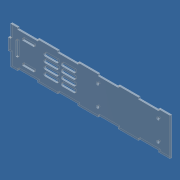
# Autodesk Inventor part: Top
Saved by Autodesk Inventor 2016 (Build 200138000, 138)
## iProperties
Created: 2016-04-03
Part Number: Top
Material: Polycarbonate, Clear
Document SubType Name: Modeling
Designer: admin
Density: 1.2 g/cm^3
Appearance: Polycarbonate - Clear
Author: admin
Autodesk Inventor part; units mm, degrees
ref_plane "YZ Plane" through (0, 0, 0) normal (1, 0, 0) x (0, 1, 0)
ref_plane "XZ Plane" through (0, 0, 0) normal (0, 1, 0) x (-1, 0, 0)
ref_plane "XY Plane" through (0, 0, 0) normal (0, 0, 1) x (1, 0, 0)
derived "Wall.ipt"
sketch "Sketch1" plane through (0, 0, 0) normal (0, 0, 1) x (1, 0, 0)
  line L0 (142.5, -22.5) -> (142.5, 22.5)
  line L1 (142.5, 22.5) -> (-137.5, 22.5)
  arc A0 (-169.3198, -9.3198) -> (-157.5, -22.5) centre (-130.5627, 13.547) ccw
  line L2 (-154.4706, 5.5294) -> (-150.935, 1.9939)
  line L3 (-150.935, 1.9939) -> (-152.2157, 0.7132)
  line L4 (-152.2157, 0.7132) -> (-150.8015, -0.701)
  line L5 (-150.8015, -0.701) -> (-149.5208, 0.5797)
  line L6 (-149.5208, 0.5797) -> (-147.3995, -1.5416)
  line L7 (-147.3995, -1.5416) -> (-145.2782, 0.5797)
  line L8 (-145.2782, 0.5797) -> (-147.3995, 2.701)
  line L9 (-147.3995, 2.701) -> (-146.1188, 3.9817)
  line L10 (-146.1188, 3.9817) -> (-147.533, 5.3959)
  line L11 (-147.533, 5.3959) -> (-148.8137, 4.1152)
  line L12 (-148.8137, 4.1152) -> (-152.3492, 7.6508)
  line L13 (-154.542, 7.7222) -> (-156.666, 9.8462) construction
  line L14 (-122.5, 22.5) -> (-122.5, 25.5)
  line L15 (-122.5, 25.5) -> (-87.5, 25.5)
  line L16 (-87.5, 25.5) -> (-87.5, 22.5)
  line L17 (-52.5, 22.5) -> (-52.5, 25.5)
  line L18 (-52.5, 25.5) -> (-17.5, 25.5)
  line L19 (-17.5, 25.5) -> (-17.5, 22.5)
  line L20 (17.5, 22.5) -> (17.5, 25.5)
  line L21 (17.5, 25.5) -> (52.5, 25.5)
  line L22 (52.5, 25.5) -> (52.5, 22.5)
  line L23 (87.5, 22.5) -> (87.5, 25.5)
  line L24 (87.5, 25.5) -> (122.5, 25.5)
  line L25 (122.5, 25.5) -> (122.5, 22.5)
  line L26 (87.5, 22.5) -> (52.5, 22.5)
  line L27 (-52.5, 22.5) -> (-87.5, 22.5)
  line L28 (-122.5, 22.5) -> (-137.5, 22.5)
  line L29 (-122.5, -22.5) -> (-122.5, -25.5)
  line L30 (-122.5, -25.5) -> (-87.5, -25.5)
  line L31 (-87.5, -25.5) -> (-87.5, -22.5)
  line L32 (-52.5, -22.5) -> (-52.5, -25.5)
  line L33 (-52.5, -25.5) -> (-17.5, -25.5)
  line L34 (-17.5, -25.5) -> (-17.5, -22.5)
  line L35 (17.5, -22.5) -> (17.5, -25.5)
  line L36 (17.5, -25.5) -> (52.5, -25.5)
  line L37 (52.5, -25.5) -> (52.5, -22.5)
  line L38 (87.5, -22.5) -> (87.5, -25.5)
  line L39 (87.5, -25.5) -> (122.5, -25.5)
  line L40 (122.5, -25.5) -> (122.5, -22.5)
  line L41 (-157.5, -22.5) -> (-122.5, -22.5)
  line L42 (-87.5, -22.5) -> (-52.5, -22.5)
  line L43 (-17.5, -22.5) -> (17.5, -22.5)
  line L44 (52.5, -22.5) -> (87.5, -22.5)
  line L45 (122.5, -22.5) -> (142.5, -22.5)
  line L46 (-1.5, 12.5) -> (-1.5, 22.5)
  line L47 (1.5, 22.5) -> (1.5, 12.5)
  line L48 (1.5, 12.5) -> (-1.5, 12.5)
  line L49 (-37.337, 0) -> (-30.889, 0) construction
  line L50 (-164.0165, -4.0165) -> (-166.1378, -1.8952)
  line L51 (-166.1378, -1.8952) -> (-161.8952, 2.3475)
  line L52 (-161.8952, 2.3475) -> (-159.7739, 0.2261)
  line L53 (-147.0459, 12.9541) -> (-149.1673, 15.0754)
  line L54 (-149.1673, 15.0754) -> (-144.9246, 19.318)
  line L55 (-144.9246, 19.318) -> (-142.8033, 17.1967)
  line L56 (-154.4706, 5.5294) -> (-159.7739, 0.2261)
  line L57 (-164.0165, -4.0165) -> (-169.3198, -9.3198)
  line L58 (-137.5, 22.5) -> (-142.8033, 17.1967)
  line L59 (-147.0459, 12.9541) -> (-152.3492, 7.6508)
  line L60 (17.5, 22.5) -> (1.5, 22.5)
  line L61 (-1.5, 22.5) -> (-17.5, 22.5)
  line L62 (131, 22.5) -> (131, 12.5)
  line L63 (131, 12.5) -> (134, 12.5)
  line L64 (134, 12.5) -> (134, 22.5)
  line L65 (122.5, 22.5) -> (131, 22.5)
  line L66 (134, 22.5) -> (142.5, 22.5)
  point P0 (0, 0)
  point P1 (142.5, 0)
  point P2 (-146.3388, -0.481)
  point P3 (2.493, 0)
  point P4 (0, -22.5)
  point P5 (1.5, -22.5)
sketch "Sketch2" plane through (0, 0, 0) normal (0, 1, 0) x (-1, 0, 0)
  line L0 (-142.5, 0) -> (137.5, 0) construction
  line L1 (-142.5, -65) -> (-142.5, 0)
  line L2 (134.5, -42.5) -> (138.5, -42.5)
  line L3 (138.5, -42.5) -> (138.5, -22.5)
  line L4 (138.5, -22.5) -> (134.5, -22.5)
  line L5 (134.5, 0) -> (134.5, -22.5)
  line L6 (134.5, -42.5) -> (134.5, -65)
  line L7 (122.5, 0) -> (122.5, -3)
  line L8 (122.5, -3) -> (87.5, -3)
  line L9 (87.5, -3) -> (87.5, 0)
  line L10 (52.5, 0) -> (52.5, -3)
  line L11 (52.5, -3) -> (17.5, -3)
  line L12 (17.5, -3) -> (17.5, 0)
  line L13 (-17.5, 0) -> (-17.5, -3)
  line L14 (-17.5, -3) -> (-52.5, -3)
  line L15 (-52.5, -3) -> (-52.5, 0)
  line L16 (-87.5, 0) -> (-87.5, -3)
  line L17 (-87.5, -3) -> (-122.5, -3)
  line L18 (-122.5, -3) -> (-122.5, 0)
  line L19 (122.5, -65) -> (122.5, -62)
  line L20 (122.5, -62) -> (87.5, -62)
  line L21 (87.5, -62) -> (87.5, -65)
  line L22 (52.5, -65) -> (52.5, -62)
  line L23 (17.5, -62) -> (17.5, -65)
  line L24 (17.5, -62) -> (52.5, -62)
  line L25 (-17.5, -65) -> (-17.5, -62)
  line L26 (-52.5, -62) -> (-52.5, -65)
  line L27 (-52.5, -62) -> (-17.5, -62)
  line L28 (-87.5, -65) -> (-87.5, -62)
  line L29 (-87.5, -62) -> (-122.5, -62)
  line L30 (-122.5, -62) -> (-122.5, -65)
  line L31 (134.5, -65) -> (122.5, -65)
  line L32 (87.5, -65) -> (52.5, -65)
  line L33 (17.5, -65) -> (-17.5, -65)
  line L34 (-52.5, -65) -> (-87.5, -65)
  line L35 (-122.5, -65) -> (-142.5, -65)
  line L36 (87.5, 0) -> (52.5, 0)
  line L37 (17.5, 0) -> (-17.5, 0)
  line L38 (-52.5, 0) -> (-87.5, 0)
  line L39 (-122.5, 0) -> (-142.5, 0)
  line L40 (134.5, 0) -> (122.5, 0)
  point P0 (0, 0)
  point P1 (138.5, -32.5)
  point P2 (-142.5, -32.5)
  dimension "d1" = 65
  dimension "d4" = 20
  dimension "d5" = 4
  dimension "d6" = 3
  dimension "d7" = 3
  constraints: 80 end point, 28 point on line, 25 perpendicular, 6 collinear, 6 horizontal, 4 vertical, 3 parallel, 2 midpoint, 1 horizontal alignment, 2 other
  measures "d1" distance of L1.start L1.end
  measures "d4" distance between parallel lines of L4 L2
  measures "d5" distance between parallel lines of L6 L3
  measures "d6" distance of L20.end L21.end
  measures "d7" distance from line of L5 point (137.5, 0)
extrude "Extrusion1" add sketch "Sketch2" along normal blind 3
sketch "Sketch4" plane through (0, 3, 0) normal (0, 1, 0) x (1, 0, 0)
  line L0 (-122.5, 45) -> (-125.5, 45)
  line L1 (-125.5, 45) -> (-125.5, 20)
  line L2 (-125.5, 20) -> (-122.5, 20)
  line L3 (-122.5, 20) -> (-122.5, 45)
  line L4 (142.5, 0) -> (142.5, 65) projected
  line L5 (142.5, 65) -> (122.5, 65) projected
  line L6 (122.5, 65) -> (122.5, 62) projected
  line L7 (122.5, 62) -> (87.5, 62) projected
  line L8 (87.5, 62) -> (87.5, 65) projected
  line L9 (87.5, 65) -> (52.5, 65) projected
  line L10 (52.5, 65) -> (52.5, 62) projected
  line L11 (52.5, 62) -> (17.5, 62) projected
  line L12 (17.5, 62) -> (17.5, 65) projected
  line L13 (17.5, 65) -> (-17.5, 65) projected
  line L14 (-17.5, 65) -> (-17.5, 62) projected
  line L15 (-17.5, 62) -> (-52.5, 62) projected
  line L16 (-52.5, 62) -> (-52.5, 65) projected
  line L17 (-52.5, 65) -> (-87.5, 65) projected
  line L18 (-87.5, 65) -> (-87.5, 62) projected
  line L19 (-87.5, 62) -> (-122.5, 62) projected
  line L20 (-122.5, 62) -> (-122.5, 65) projected
  line L21 (-122.5, 65) -> (-134.5, 65) projected
  line L22 (-134.5, 65) -> (-134.5, 42.5) projected
  line L23 (-134.5, 42.5) -> (-138.5, 42.5) projected
  line L24 (-138.5, 42.5) -> (-138.5, 22.5) projected
  line L25 (-138.5, 22.5) -> (-134.5, 22.5) projected
  line L26 (-134.5, 22.5) -> (-134.5, 0) projected
  line L27 (-134.5, 0) -> (-122.5, 0) projected
  line L28 (-122.5, 0) -> (-122.5, 3) projected
  line L29 (-122.5, 3) -> (-87.5, 3) projected
  line L30 (-87.5, 3) -> (-87.5, 0) projected
  line L31 (-87.5, 0) -> (-52.5, 0) projected
  line L32 (-52.5, 0) -> (-52.5, 3) projected
  line L33 (-52.5, 3) -> (-17.5, 3) projected
  line L34 (-17.5, 3) -> (-17.5, 0) projected
  line L35 (-17.5, 0) -> (17.5, 0) projected
  line L36 (17.5, 0) -> (17.5, 3) projected
  line L37 (17.5, 3) -> (52.5, 3) projected
  line L38 (52.5, 3) -> (52.5, 0) projected
  line L39 (52.5, 0) -> (87.5, 0) projected
  line L40 (87.5, 0) -> (87.5, 3) projected
  line L41 (87.5, 3) -> (122.5, 3) projected
  line L42 (122.5, 3) -> (122.5, 0) projected
  line L43 (122.5, 0) -> (142.5, 0) projected
  line L44 (-122.5, 62) -> (-122.5, 65) projected
  line L45 (-119.5, 86.0571) -> (-119.5, -26.187) construction
  line L46 (-117, 86.0571) -> (-117, -26.187) construction
  line L47 (-114, 53.2887) -> (-114, 7.6341) construction
  line L48 (-114, 53) -> (-94, 53)
  line L49 (-94, 53) -> (-94, 50)
  line L50 (-94, 50) -> (-114, 50)
  line L51 (-114, 50) -> (-114, 53)
  line L52 (-114, 15) -> (-94, 15)
  line L53 (-94, 15) -> (-94, 12)
  line L54 (-94, 12) -> (-114, 12)
  line L55 (-114, 12) -> (-114, 15)
  line L56 (-94.6514, 32.5) -> (-74.3553, 32.5) construction
  point P0 (0, 0)
  point P1 (-138.5, 32.5)
  point P2 (-122.5, 32.5)
  dimension "d20" = 25
  dimension "d24" = 265
  dimension "d25" = 3
  dimension "d27" = 2.5
  dimension "d28" = 3
  dimension "d29" = 35
  dimension "d30" = 20
  constraints: 32 end point, 6 parallel, 4 horizontal, 3 collinear, 3 equal length, 3 horizontal alignment, 3 perpendicular, 3 vertical, 2 midpoint, 1 point on line, 1 other
  measures "d20" distance between parallel lines of L2 L0
  measures "d24" distance between parallel lines of L4 L3
  measures "d25" distance between parallel lines of L45 L3
  measures "d27" distance between parallel lines of L45 L46
  measures "d28" distance between parallel lines of L47 L46
  measures "d29" distance between parallel lines of L52 L50
  measures "d30" distance of L53.end L54.end
extrude "Extrusion3" cut sketch "Sketch4" against normal up to next contours L3 L2 L1 L0 | L48 L49 L50 L51 | L52 L53 L54 L55
sketch "Sketch3" plane through (0, 3, 0) normal (0, 1, 0) x (1, 0, 0)
  arc A0 (-74.5, 19.5) -> (-74.5, 14.5) centre (-74.5, 17) ccw
  arc A1 (-54.5, 14.5) -> (-54.5, 19.5) centre (-54.5, 17) ccw
  line L0 (-74.5, 19.5) -> (-54.5, 19.5)
  line L1 (-74.5, 14.5) -> (-54.5, 14.5)
  line L2 (-122.5, 3) -> (-87.5, 3) projected
  line L3 (-134.5, 22.5) -> (-134.5, 0) projected
  point P0 (0, 0)
  dimension "d8" = 5
  dimension "d9" = 20
  dimension "d10" = 14
  dimension "d11" = 60
  constraints: 4 end point, 4 point on circle, 3 tangent, 2 centre point, 1 equal radius, 1 horizontal, 1 horizontal alignment
  measures "d8" diameter of A0
  measures "d9" distance of A1.centre A0.centre
  measures "d10" distance from line of L2 A0.centre
  measures "d11" distance from line of L3 A0.centre
extrude "Extrusion2" cut sketch "Sketch3" against normal blind 3
pattern_linear "Rectangular Pattern1" count 2 spacing 30 along (1, 0, 0) count 4 spacing 10 along (0, 0, -1) of "Extrusion2"
sketch "Sketch5" plane through (0, 0, 0) normal (0, -1, 0) x (1, 0, 0)
  line L0 (4.9906, -32.5) -> (36.8518, -32.5) construction
  line L1 (142.5, 0) -> (142.5, -65) construction
  point P0 (0, 0)
  point P1 (16.5, -15)
  point P2 (16.5, -50)
  point P3 (121.5, -15)
  point P4 (121.5, -50)
  point P5 (142.5, -32.5)
  dimension "d31" = 35
  dimension "d32" = 16.5
  dimension "d33" = 105
  constraints: 2 end point, 2 horizontal alignment, 2 vertical alignment, 1 horizontal, 1 midpoint, 1 point on line, 1 symmetric about line
  measures "d31" distance of point (16.5, -50) point (16.5, -15)
  measures "d32" horizontal distance of point (16.5, -15) point (0, 0)
  measures "d33" distance of point (121.5, -15) point (16.5, -15)
hole "Hole1" at (16.5, 0, -15) at (16.5, 0, -50) at (121.5, 0, -15) at (121.5, 0, -50) direction (0, 1, 0) diameter 3 end through all countersink diameter 5 countersink angle 90
body "Solid1"
